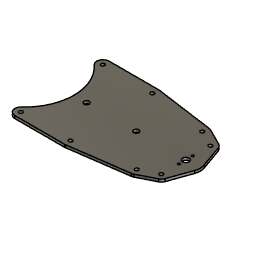
Gearbox Plate Top v9 (Autodesk Fusion 360 design; units mm, degrees)
Autodesk Fusion 360 part; units mm, degrees
sketch "Sketch1" plane through (0, 0, 0) normal (0, 0, 1) x (1, 0, 0)
  circle A0 centre (0, 0) radius 4
  line L0 (0, 0) -> (-60.5, 0) construction
  line L1 (-60.5, 0) -> (-121, 0) construction
  circle A1 centre (-60.5, 0) radius 3.15
  circle A2 centre (-121, 0) radius 3.15
  circle A3 centre (-60.5, 0) radius 47 construction
  circle A4 centre (-121, 0) radius 47 construction
  circle A5 centre (0, 0) radius 17.5
  circle A6 centre (-60.5, 0) radius 17 construction
  circle A7 centre (0, 0) radius 12.5 construction
  circle A8 centre (0, 30) radius 2.25
  circle A9 centre (0, -30) radius 2.25
  circle A10 centre (0, 30) radius 6 construction
  circle A11 centre (0, -30) radius 6 construction
  line L2 (-90.75, 0) -> (-90.75, 50) construction
  circle A12 centre (-90.75, 50) radius 7.5
  circle A13 centre (-90.75, 50) radius 2.25
  line L3 (-90.75, 0) -> (-90.75, -50) construction
  circle A14 centre (-90.75, -50) radius 7.5
  circle A15 centre (-90.75, -50) radius 2.25
  line L4 (-121, 0) -> (-151.25, 0) construction
  line L5 (-151.25, 0) -> (-151.25, 50) construction
  circle A16 centre (-151.25, 50) radius 7.5
  circle A17 centre (-151.25, 50) radius 2.25
  line L6 (-151.25, 0) -> (-151.25, -50) construction
  circle A18 centre (-151.25, -50) radius 7.5
  circle A19 centre (-151.25, -50) radius 2.25
  circle A20 centre (-20, 40) radius 7.5
  line L7 (-20, 40) -> (-20, 0) construction
  line L8 (-20, 0) -> (-20, -40) construction
  circle A21 centre (-20, -40) radius 7.5
  circle A22 centre (-20, -40) radius 2.25
  circle A23 centre (-20, 40) radius 2.25
  line L9 (-89.7004, -57.4262) -> (-18.9504, -47.4262)
  circle A24 centre (0, -30) radius 7.5
  circle A25 centre (0, 30) radius 7.5
  line L10 (-89.7004, 57.4262) -> (-18.9504, 47.4262)
  circle A26 centre (-196.5959, 0) radius 60
  line L11 (-16.6459, 46.7082) -> (3.3541, 36.7082)
  line L12 (7.0711, 32.5) -> (16.4992, 5.8333)
  line L13 (7.0711, -32.5) -> (16.4992, -5.8333)
  line L14 (-16.6459, -46.7082) -> (3.3541, -36.7082)
  circle A27 centre (-121, 86.6222) radius 40
  line L15 (-151.25, -57.5) -> (-90.75, -57.5)
  line L16 (-160.1233, -61.9813) -> (16.4992, -61.9813) construction
  circle A28 centre (0, 0) radius 8.5 construction
  circle A29 centre (0, 8.5) radius 1.4
  circle A30 centre (0, -8.5) radius 1.4
  line L17 (-151.25, 57.5) -> (-90.75, 57.5)
  dimension "d1" = 8
  dimension "d2" = 60.5
  dimension "d4" = 60.5
  dimension "d6" = 6.3
  dimension "d7" = 6.3
  dimension "d8" = 94
  dimension "d9" = 94
  dimension "d10" = 35
  dimension "d11" = 34
  dimension "d12" = 25
  dimension "d13" = 4.5
  dimension "d14" = 4.5
  dimension "d15" = 60
  dimension "d16" = 12
  dimension "d17" = 12
  dimension "d18" = 15
  dimension "d19" = 50
  dimension "d20" = 4.5
  dimension "d21" = 15
  dimension "d22" = 4.5
  dimension "d23" = 30.25
  dimension "d24" = 15
  dimension "d25" = 4.5
  dimension "d26" = 15
  dimension "d27" = 4.5
  dimension "d28" = 15
  dimension "d29" = 40
  dimension "d30" = 20
  dimension "d31" = 15
  dimension "d32" = 4.5
  dimension "d33" = 4.5
  dimension "d34" = 15
  dimension "d35" = 15
  dimension "d36" = 120
  dimension "d37" = 80
  dimension "d44" = 17
  dimension "d45" = 2.8
  dimension "d46" = 2.8
  constraint coincident A0.centre L0.start
  constraint horizontal L0
  constraint horizontal L1
  constraint coincident L0.end L1.start
  constraint coincident L1.end A2.centre
  constraint concentric A1 A3
  constraint concentric A2 A4
  constraint vertical A0.centre A8.centre
  constraint vertical A0.centre A9.centre
  constraint symmetric L0 A8 A9
  constraint concentric A8 A10
  constraint concentric A9 A11
  constraint midpoint L1 L2.start
  constraint perpendicular L1 L2
  constraint coincident L2.end A12.centre
  constraint concentric A12 A13
  constraint perpendicular L1 L3
  constraint equal L2 L3
  constraint coincident L3.end A14.centre
  constraint concentric A14 A15
  constraint parallel L1 L4
  constraint perpendicular L4 L5
  constraint equal L2 L5
  constraint coincident L5.end A16.centre
  constraint concentric A16 A17
  constraint perpendicular L4 L6
  constraint equal L3 L6
  constraint coincident L6.end A18.centre
  constraint concentric A18 A19
  constraint coincident A20.centre L7.start
  constraint coincident L0 L7.end
  constraint perpendicular L0 L7
  constraint perpendicular L0 L8
  constraint coincident L8.end A21.centre
  constraint concentric A21 A22
  constraint concentric A20 A23
  constraint equal L7 L8
  constraint coincident A14 L9.start
  constraint coincident A21 L9.end
  constraint tangent A21 L9
  constraint tangent A14 L9
  constraint concentric A11 A24
  constraint concentric A10 A25
  constraint coincident A12 L10.start
  constraint coincident A20 L10.end
  constraint tangent A20 L10
  constraint tangent A12 L10
  constraint tangent A16 A26
  constraint tangent A18 A26
  constraint coincident A20 L11.start
  constraint coincident A25 L11.end
  constraint tangent A25 L11
  constraint coincident A25 L12.start
  constraint coincident A5 L12.end
  constraint tangent A5 L12
  constraint coincident A24 L13.start
  constraint coincident A5 L13.end
  constraint tangent A5 L13
  constraint coincident A21 L14.start
  constraint coincident A24 L14.end
  constraint tangent A24 L14
  constraint tangent A21 L14
  constraint tangent A24 L13
  constraint tangent A25 L12
  constraint tangent A20 L11
  constraint tangent A12 A27
  constraint tangent A16 A27
  constraint coincident A18 L15.start
  constraint coincident A14 L15.end
  constraint tangent A14 L15
  constraint tangent A18 L15
  constraint horizontal L16
  constraint concentric A5 A28
  constraint coincident A28 A29.centre
  constraint coincident A28 A30.centre
  constraint vertical A0.centre A29.centre
  constraint vertical A0.centre A30.centre
  constraint coincident A16 L17.start
  constraint coincident A12 L17.end
  constraint tangent A12 L17
  constraint tangent A16 L17
  measures "d1" diameter of A0
  measures "d2" distance of A0.centre L0.end
  measures "d4" distance of L0.end L1.end
  measures "d6" diameter of A1
  measures "d7" diameter of A2
  measures "d8" diameter of A3
  measures "d9" diameter of A4
  measures "d10" diameter of A5
  measures "d11" diameter of A6
  measures "d12" diameter of A7
  measures "d13" diameter of A8
  measures "d14" diameter of A9
  measures "d15" distance of A8.centre A9.centre
  measures "d16" diameter of A10
  measures "d17" diameter of A11
  measures "d18" diameter of A12
  measures "d19" distance of L2.start L2.end
  measures "d20" diameter of A13
  measures "d21" diameter of A14
  measures "d22" diameter of A15
  measures "d23" distance of L1.end L4.end
  measures "d24" diameter of A16 A1
  measures "d25" diameter of A17 A1
  measures "d26" diameter of A18 A1
  measures "d27" diameter of A19 A1
  measures "d28" diameter of A20
  measures "d29" distance of A20.centre L7.end
  measures "d30" distance of A0.centre L7.end
  measures "d31" diameter of A21 A1
  measures "d32" diameter of A22 A1
  measures "d33" diameter of A23
  measures "d34" diameter of A24
  measures "d35" diameter of A25
  measures "d36" diameter of A26
  measures "d37" diameter of A27
  measures "d44" diameter of A28
  measures "d45" diameter of A29
  measures "d46" diameter of A30
extrude "Extrude1" add sketch "Sketch1" along normal blind 3.175 contours A5 | A5 A12 A14 A16 A18 A20 A21 L9 A24 A25 L10 A26 L11 L12 L13 L14 A27 L15 | A25 | A24 | A20 | A21 | A12 | A14 | A12 A27 L17 | A27 L17 | A18 | A16 | A16 A27 L17 picked at (-127.9955, 54.7116)
ref_plane "WorkPlane1" through (-70.7689, 0, 3.175) normal (0, 0, 1) x (1, 0, 0)
sketch "Sketch2" plane through (0, 0, 3.175) normal (0, 0, 1) x (1, 0, 0)
  circle A0 centre (-90.75, -50) radius 2.25
  circle A1 centre (0, 30) radius 2.25
  circle A2 centre (-151.25, -50) radius 2.25
  circle A3 centre (0, -30) radius 2.25
  circle A4 centre (0, 0) radius 4
  circle A5 centre (0, 8.5) radius 1.4
  circle A6 centre (0, -8.5) radius 1.4
  circle A7 centre (-20, -40) radius 2.25
  circle A8 centre (-90.75, 50) radius 2.25
  circle A9 centre (-20, 40) radius 2.25
  circle A10 centre (-151.25, 50) radius 2.25
  circle A11 centre (-60.5, 0) radius 3.15
  circle A12 centre (-121, 0) radius 3.15
  line L0 (-151.25, -57.5) -> (-90.75, -57.5)
  arc A13 (-156.2884, -44.4444) -> (-151.25, -57.5) centre (-151.25, -50) ccw
  arc A14 (-156.2884, -44.4444) -> (-156.2884, 44.4444) centre (-196.5959, 0) ccw
  arc A15 (-151.25, 57.5) -> (-156.2884, 44.4444) centre (-151.25, 50) ccw
  line L1 (-151.25, 57.5) -> (-90.75, 57.5)
  arc A16 (-89.7004, 57.4262) -> (-90.75, 57.5) centre (-90.75, 50) ccw
  line L2 (-89.7004, 57.4262) -> (-18.9504, 47.4262)
  arc A17 (-16.6459, 46.7082) -> (-18.9504, 47.4262) centre (-20, 40) ccw
  line L3 (-16.6459, 46.7082) -> (3.3541, 36.7082)
  arc A18 (7.0711, 32.5) -> (3.3541, 36.7082) centre (0, 30) ccw
  line L4 (7.0711, 32.5) -> (16.4992, 5.8333)
  arc A19 (16.4992, -5.8333) -> (16.4992, 5.8333) centre (0, 0) ccw
  line L5 (7.0711, -32.5) -> (16.4992, -5.8333)
  arc A20 (3.3541, -36.7082) -> (7.0711, -32.5) centre (0, -30) ccw
  line L6 (-16.6459, -46.7082) -> (3.3541, -36.7082)
  arc A21 (-18.9504, -47.4262) -> (-16.6459, -46.7082) centre (-20, -40) ccw
  line L7 (-89.7004, -57.4262) -> (-18.9504, -47.4262)
  arc A22 (-90.75, -57.5) -> (-89.7004, -57.4262) centre (-90.75, -50) ccw
equation "d2 = distBetweenGears"
equation "distBetweenGears = 60.5 mm"
equation "d4 = distBetweenGears"
equation "acrylicRoundHoleSize = 6.3 mm"
equation "d6 = acrylicRoundHoleSize"
equation "d7 = acrylicRoundHoleSize"
equation "d13 = WoodScrewHoleSize"
equation "d14 = WoodScrewHoleSize"
equation "d20 = WoodScrewHoleSize"
equation "d22 = WoodScrewHoleSize"
equation "d23 = distBetweenGears / 2"
equation "d25 = WoodScrewHoleSize"
equation "d27 = WoodScrewHoleSize"
equation "d32 = WoodScrewHoleSize"
equation "d33 = WoodScrewHoleSize"
equation "WoodScrewHoleSize = 4.5 mm"
